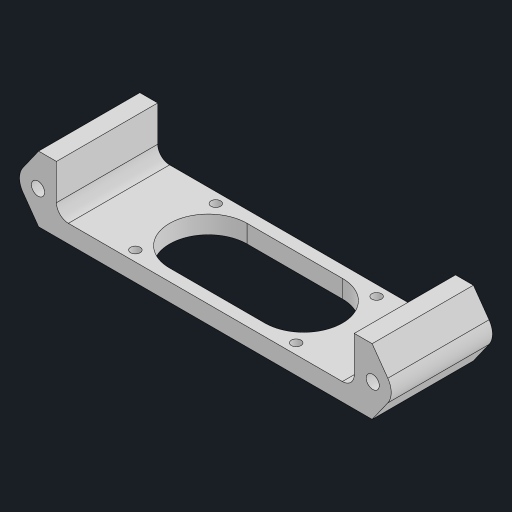
# Autodesk Inventor part: Ultrasonic_holder
Saved by Autodesk Inventor 2023 (Build 270158000, 158)
## iProperties
Created: 2022-06-21
Part Number: Ultrasonic_holder
Material: 一般
Document SubType Name: Modeling
Designer: legot
Density: 1 g/cm^3
Appearance: 既定
Author: legot
Autodesk Inventor part; units mm, degrees
ref_plane "YZ Plane" through (0, 0, 0) normal (1, 0, 0) x (0, 1, 0)
ref_plane "XZ Plane" through (0, 0, 0) normal (0, 1, 0) x (-1, 0, 0)
ref_plane "XY Plane" through (0, 0, 0) normal (0, 0, 1) x (1, 0, 0)
sketch "スケッチ1" plane through (0, 0, 0) normal (0, 1, 0) x (-1, 0, 0)
  line L0 (0, 6.75) -> (-13.5, 6.75) construction
  line L1 (-13.5, 6.75) -> (-13.5, -6.75) construction
  line L2 (-13.5, -6.75) -> (0, -6.75) construction
  line L3 (0, -6.75) -> (0, 6.75) construction
  circle A0 centre (-8, 0) radius 6.5
  line L4 (0, 8.5) -> (-25, 8.5)
  line L5 (-25, 8.5) -> (-25, -8.5)
  line L6 (-25, -8.5) -> (0, -8.5)
  line L7 (0, -8.5) -> (0, 8.5)
  line L8 (-25, 8.5) -> (-27.8, 8.5)
  line L9 (-27.8, 8.5) -> (-27.8, -8.5)
  line L10 (-27.8, -8.5) -> (-25, -8.5)
  line L11 (-25, -8.5) -> (-25, 8.5)
  line L12 (0, 6.5) -> (-8, 6.5)
  line L13 (0, -6.5) -> (-8, -6.5)
  point P0 (0, 0)
  point P1 (0, 0)
  dimension "d0" = 13.5
  dimension "d1" = 13.5
  dimension "d2" = 8
  dimension "d3" = 13
  dimension "d4" = 17
  dimension "d5" = 25
  dimension "d6" = 2.8
  constraints: 28 end point, 6 parallel, 4 horizontal, 4 perpendicular, 3 coincident, 2 midpoint, 2 point on circle, 2 point on line, 2 tangent, 1 centre point, 1 collinear, 1 horizontal alignment
  measures "d0" distance of L2.end L0.start
  measures "d1" distance of L0.start L0.end
  measures "d2" distance of A0.centre point (0, 0)
  measures "d3" diameter of A0
  measures "d4" distance of L6.end L4.start
  measures "d5" distance of L5.end L6.end
  measures "d6" distance of L9.end L10.end
extrude "押し出し1" add sketch "スケッチ1" along normal blind 3 contours A0 L13 L7 L6 L5 L4 L12
hole "穴1" at (13.5, 0, -6.75) at (13.5, 0, 6.75) direction (0, 1, 0) diameter 1.6 end through all clearance for "Flat Head Machine Screw (82)" size "#0" standard "Ansi Unified Screw Threads"
sketch "スケッチ2" plane through (0, 0, 8.5) normal (0, 0, 1) x (1, 0, 0)
  line L0 (25, 0) -> (25, 3) projected
  line L1 (0, 3) -> (25, 3) projected
  line L2 (25, 0) -> (28, 0)
  line L3 (28, 0) -> (28, 11) construction
  line L4 (28, 11) -> (25, 11)
  line L5 (25, 11) -> (25, 0)
  circle A0 centre (28.1, 5.5) radius 1.1
  arc A1 (30.6287, 7.2932) -> (30.6287, 3.7068) centre (28.1, 5.5) ccw construction
  line L6 (28, 11) -> (30.6287, 7.2932)
  line L7 (28, 0) -> (30.6287, 3.7068)
  arc A2 (30.6287, 3.7068) -> (30.6287, 7.2932) centre (28.1, 5.5) ccw
  dimension "d9" = 2.2
  dimension "d10" = 3
  dimension "d12" = 8
  dimension "d13" = 6.2
  constraints: 12 end point, 4 point on circle, 3 centre point, 3 tangent, 2 parallel, 1 coincident, 1 equal length, 1 horizontal, 1 perpendicular
  measures "d9" diameter of A0
  measures "d10" distance of L0.start L2.end
  measures "d12" distance between parallel lines of L4 L1
  measures "d13" diameter of A1
extrude "押し出し2" add sketch "スケッチ2" against normal up to surface (17 mm away)
fillet "フィレット1" radius 2 1 edges at (25, 3, 0)
mirror "ミラー1" about plane through (0, 0, -8.5) normal (-1, 0, 0) of "押し出し1", "穴1", "押し出し2", "フィレット1"
